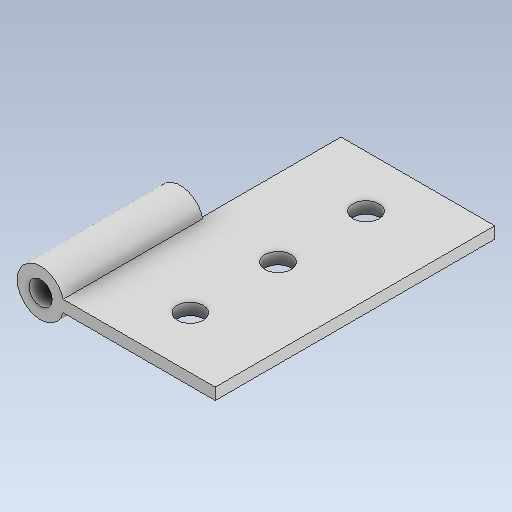
# Autodesk Inventor part: leaf
Saved by Autodesk Inventor 2020 (Build 240168000, 168)
## iProperties
Created: 2021-11-11
Part Number: leaf
Material: Generic
Document SubType Name: Modeling
Designer: 17185
Density: 1 g/cm^3
Appearance: Default
Author: 17185
Autodesk Inventor part; units mm, degrees
ref_plane "YZ Plane" through (0, 0, 0) normal (1, 0, 0) x (0, 1, 0)
ref_plane "XZ Plane" through (0, 0, 0) normal (0, 1, 0) x (-1, 0, 0)
ref_plane "XY Plane" through (0, 0, 0) normal (0, 0, 1) x (1, 0, 0)
sketch "Sketch1" plane through (0, 0, 0) normal (0, 1, 0) x (-1, 0, 0)
  line L0 (20.955, 38.1) -> (-20.955, 38.1)
  line L1 (-20.955, 38.1) -> (-20.955, -38.1)
  line L2 (-20.955, -38.1) -> (20.955, -38.1)
  line L3 (20.955, -38.1) -> (20.955, 38.1)
  line L4 (20.955, 38.1) -> (-20.955, -38.1) construction
  line L5 (-20.955, 38.1) -> (20.955, -38.1) construction
  circle A0 centre (0, -23.962) radius 3.556
  circle A1 centre (0, 0) radius 3.556
  line L6 (10.0795, 23.962) -> (-10.0795, 23.962) construction
  line L7 (-10.0795, 23.962) -> (-10.0795, -23.962) construction
  line L8 (-10.0795, -23.962) -> (10.0795, -23.962) construction
  line L9 (10.0795, -23.962) -> (10.0795, 23.962) construction
  line L10 (10.0795, 23.962) -> (-10.0795, -23.962) construction
  line L11 (-10.0795, 23.962) -> (10.0795, -23.962) construction
  circle A2 centre (0, 23.962) radius 3.556
  dimension "d0" = 76.2
  dimension "d1" = 41.91
  dimension "d2" = 7.112
  dimension "d3" = 7.112
  dimension "d4" = 7.112
  constraints: 24 end point, 5 midpoint, 4 parallel, 3 centre point, 2 horizontal, 2 perpendicular, 1 coincident
  measures "d0" distance of L0.end L1.end
  measures "d1" distance of L1.end L2.end
  measures "d2" diameter of A0
  measures "d3" diameter of A1
  measures "d4" diameter of A2
extrude "Extrusion1" add sketch "Sketch1" along normal blind 3.175
sketch "Sketch2" plane through (-20.955, 0, 38.1) normal (0, 0, 1) x (1, 0, 0)
  circle A0 centre (-5.715, 1.5875) radius 3.175
  line L0 (0, 0) -> (0, 3.175) projected
  circle A1 centre (-5.715, 1.5875) radius 6.35
  point P0 (20.955, 0)
  dimension "d7" = 6.35
  dimension "d8" = 5.715
  dimension "d11" = 12.7
  constraints: 2 centre point, 1 coincident
  measures "d7" diameter of A0
  measures "d8" distance from line of L0 A0.centre
  measures "d11" diameter of A1
extrude "Extrusion2" add sketch "Sketch2" against normal blind 38.1
body "Solid1"
